mtg (Autodesk Fusion 360 design; units mm, degrees)
Autodesk Fusion 360 part; units mm, degrees
sketch "Sketch3" plane through (0, 0, 0) normal (0, 1, 0) x (1, 0, 0)
  line L0 (0, 0) -> (0, -81.278)
  line L1 (0, 0) -> (0, 74.0631)
  line L2 (0, -81.278) -> (-6.1094, -18.3379)
  line L3 (-10.0828, -18.2688) -> (-15.5505, -59.5807)
  line L4 (-17.7316, -59.5801) -> (-23.6198, -14.8734)
  line L5 (-27.968, -14.7811) -> (-33.054, -43.818)
  line L6 (-35.0344, -43.7421) -> (-38.7202, -5.7707)
  spline S0 degree 5 poles (-36.9684, -2.7465) (-33.1615, -1.0281) (-25.8647, 2.9065) (-16.9676, 9.9277) (-8.9477, 21.1772) (-3.3444, 37.3639) (-1.0644, 51.6095) (-0.2181, 62.6916) (-0.0129, 70.245) (0, 74.0631) knots 0.018395 0.018395 0.018395 0.018395 0.018395 0.018395 0.2 0.4 0.6 0.8 1 1 1 1 1 1
  arc A0 (-35.0344, -43.7421) -> (-33.054, -43.818) centre (-34.039, -43.6455) ccw
  arc A1 (-17.7316, -59.5801) -> (-15.5505, -59.5807) centre (-16.641, -59.4364) ccw
  arc A2 (-6.1094, -18.3379) -> (-10.0828, -18.2688) centre (-8.1001, -18.5312) ccw
  arc A3 (-23.6198, -14.8734) -> (-27.968, -14.7811) centre (-25.801, -15.1607) ccw
  arc A4 (-36.9684, -2.7465) -> (-38.7202, -5.7707) centre (-35.7342, -5.4808) ccw
  line L7 (0, -81.278) -> (6.1094, -18.3379)
  line L8 (27.968, -14.7811) -> (33.054, -43.818)
  arc A5 (10.0828, -18.2688) -> (6.1094, -18.3379) centre (8.1001, -18.5312) ccw
  line L9 (10.0828, -18.2688) -> (15.5505, -59.5807)
  arc A6 (15.5505, -59.5807) -> (17.7316, -59.5801) centre (16.641, -59.4364) ccw
  line L10 (17.7316, -59.5801) -> (23.6198, -14.8734)
  arc A7 (27.968, -14.7811) -> (23.6198, -14.8734) centre (25.801, -15.1607) ccw
  line L11 (35.0344, -43.7421) -> (38.7202, -5.7707)
  arc A8 (38.7202, -5.7707) -> (36.9684, -2.7465) centre (35.7342, -5.4808) ccw
  spline S1 degree 5 poles (36.9684, -2.7465) (33.1615, -1.0281) (25.8647, 2.9065) (16.9676, 9.9277) (8.9477, 21.1772) (3.3444, 37.3639) (1.0644, 51.6095) (0.2181, 62.6916) (0.0129, 70.245) (0, 74.0631) knots 0.018395 0.018395 0.018395 0.018395 0.018395 0.018395 0.2 0.4 0.6 0.8 1 1 1 1 1 1
  line L12 (-47.6355, -7.5614) -> (-26.3013, 2.0685)
  line L13 (-0.0348, 63.7164) -> (0.0348, 84.4098)
  line L14 (47.6355, -7.5614) -> (26.3013, 2.0685)
  line L15 (0.0348, 63.7164) -> (-0.0348, 84.4098)
  arc A9 (33.054, -43.818) -> (35.0344, -43.7421) centre (34.039, -43.6455) ccw
  spline S2 degree 3 poles (38.557, 0.773) (30.0117, 4.6302) (23.8691, 9.367) (19.2877, 14.8219) (14.4064, 20.6339) (11.2191, 27.3028) (8.9567, 34.59) (6.553, 42.3319) (5.1997, 50.7297) (4.4743, 59.4637) (4.078, 64.2349) (3.8781, 69.1112) (3.8613, 74.0761) (2.5742, 456.4042) (1.2871, 838.7324) (0, 1221.0606) knots 0.018395 0.018395 0.018395 0.018395 0.275644 0.275644 0.275644 0.549733 0.549733 0.549733 0.840926 0.840926 0.840926 1 1 1 13.016372 13.016372 13.016372 13.016372
  spline S3 degree 3 poles (-38.557, 0.773) (-30.0117, 4.6302) (-23.8691, 9.367) (-19.2877, 14.8219) (-14.4064, 20.6339) (-11.2191, 27.3028) (-8.9567, 34.59) (-6.553, 42.3319) (-5.1997, 50.7297) (-4.4743, 59.4637) (-4.078, 64.2349) (-3.8781, 69.1112) (-3.8613, 74.0761) (-2.5742, 456.4042) (-1.2871, 838.7324) (0, 1221.0606) knots 0.018395 0.018395 0.018395 0.018395 0.275644 0.275644 0.275644 0.549733 0.549733 0.549733 0.840926 0.840926 0.840926 1 1 1 13.016372 13.016372 13.016372 13.016372
  arc A10 (-38.557, 0.773) -> (-42.5635, -6.1437) centre (-35.7342, -5.4808) ccw
  line L16 (-38.8777, -44.1152) -> (-42.5635, -6.1437)
  arc A11 (-38.8777, -44.1152) -> (-29.2506, -44.4843) centre (-34.039, -43.6455) ccw
  line L17 (-26.0335, -26.1179) -> (-29.2506, -44.4843)
  line L18 (-21.5599, -60.0843) -> (-26.0335, -26.1179)
  arc A12 (-21.5599, -60.0843) -> (-11.7225, -60.0874) centre (-16.641, -59.4364) ccw
  line L19 (-8.3845, -34.8668) -> (-11.7225, -60.0874)
  line L20 (0, -121.2453) -> (-8.3845, -34.8668)
  line L21 (0, -121.2453) -> (8.3845, -34.8668)
  line L22 (8.3845, -34.8668) -> (11.7225, -60.0874)
  arc A13 (11.7225, -60.0874) -> (21.5599, -60.0843) centre (16.641, -59.4364) ccw
  line L23 (21.5599, -60.0843) -> (26.0335, -26.1179)
  line L24 (26.0335, -26.1179) -> (29.2506, -44.4843)
  arc A14 (29.2506, -44.4843) -> (38.8777, -44.1152) centre (34.039, -43.6455) ccw
  line L25 (38.8777, -44.1152) -> (42.5635, -6.1437)
  arc A15 (42.5635, -6.1437) -> (38.557, 0.773) centre (35.7342, -5.4808) ccw
  dimension "d3" = 81.278
  dimension "d4" = 1
  dimension "d5" = 1.1
  dimension "d6" = 2
  dimension "d7" = 2.2
  dimension "d8" = 3
  dimension "d9" = 3.8614
  constraint coincident L0.start L1.start
  constraint vertical L0
  constraint parallel L0 L1
  constraint tangent L5 A0
  constraint tangent L6 A0
  constraint tangent L3 A1
  constraint tangent L4 A1
  constraint tangent L2 A2
  constraint tangent L3 A2
  constraint tangent L4 A3
  constraint tangent L5 A3
  constraint tangent L6 A4
  constraint tangent S0 A4
  constraint midpoint S0.start L12
  constraint midpoint L1.end L13
  constraint symmetric L2.start L0 L7.start
  constraint symmetric L0 L1.end S0.end
  constraint symmetric L0 L5.end L8.end
  constraint symmetric L0 L6.start L11.start
  constraint symmetric L0 A0 A9
  constraint symmetric L0 L3.end L9.end
  constraint symmetric L0 L4.start A6.end
  constraint symmetric L0 A1 A6
  constraint symmetric L0 L2.end L7.end
  constraint symmetric L0 L3.start A5.start
  constraint symmetric L0 A2 A5
  constraint symmetric L0 L4.end L10.end
  constraint symmetric L0 L5.start L8.start
  constraint symmetric L0 A3 A7
  constraint symmetric L0 S0.start A8.end
  constraint symmetric L0 A4 A8
  constraint symmetric L0 L6.end L11.end
  constraint symmetric L0 L12.start L14.start
  constraint symmetric L0 L12.end L14.end
  constraint symmetric L0 L13.start L15.start
  constraint symmetric L0 L13.end L15.end
  measures "d3" distance of L0.start L0.end
  measures "d4" radius of A0
  measures "d5" radius of A1
  measures "d6" radius of A2
  measures "d7" radius of A3
  measures "d8" radius of A4
extrude "Extrude1" add sketch "Sketch3" along normal blind 2 contours L0 L1 L7 L8 A5 L9 A6 L10 A7 L11 A8 S1 A9 | L0 L1 L2 L3 L4 L5 L6 S0 A0 A1 A2 A3 A4
extrude "Extrude2" add sketch "Sketch3" along normal blind 6 contours L2 L3 L4 L5 L6 A0 A1 A2 A3 A4 L7 L8 A5 L9 A6 L10 A7 L11 A8 L12 L14 A9 A10 L16 A11 L17 L18 A12 L19 L20 L21 L22 A13 L23 L24 A14 L25 A15 | S0 S1 L12 L14 S2 S3 A10 A15
fillet "Fillet3" radius 1 2 edges at (0, 4, 81.278) (0, 4, -74.0631)
fillet "Fillet4" radius 4.7 2 edges at (0, 3, 121.2453) (0, 3, -1221.0606)
fillet "Fillet5" radius 0.5 4 edges at (26.0335, 3, 26.1179) (8.3845, 3, 34.8668) (-8.3845, 3, 34.8668) (-26.0335, 3, 26.1179)
fillet "Fillet1" [suppressed]
fillet "Fillet2" [suppressed]
